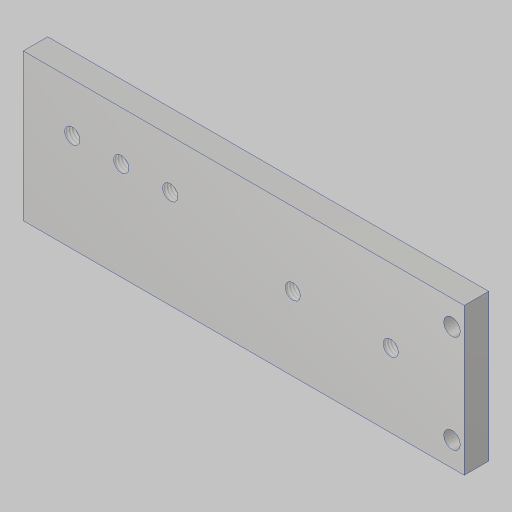
# Autodesk Inventor part: EL2-014
Saved by Autodesk Inventor 2023.5 (Build 275446000, 446)
## iProperties
Created: 2025-01-21
Part Number: EL2-014
Material: Aluminum 6061
Document SubType Name: Modeling
Designer: slick
Density: 2.7 g/cm^3
Appearance: Aluminum - Flat
Author: slick
Autodesk Inventor part; units mm, degrees
ref_plane "YZ Plane" through (0, 0, 0) normal (1, 0, 0) x (0, 1, 0)
ref_plane "XZ Plane" through (0, 0, 0) normal (0, 1, 0) x (-1, 0, 0)
ref_plane "XY Plane" through (0, 0, 0) normal (0, 0, 1) x (1, 0, 0)
sketch "Sketch1" plane through (0, 0, 0) normal (0, 0, 1) x (1, 0, 0)
  line L0 (57.15, -19.05) -> (-57.15, -19.05)
  line L1 (-57.15, -19.05) -> (-57.15, 19.05)
  line L2 (-57.15, 19.05) -> (57.15, 19.05)
  line L3 (57.15, 19.05) -> (57.15, -19.05)
  line L4 (57.15, -19.05) -> (-57.15, 19.05) construction
  line L5 (-57.15, -19.05) -> (57.15, 19.05) construction
  point P0 (0, 0)
  dimension "d0" = 114.3
  dimension "d1" = 38.1
  constraints: 12 end point, 2 midpoint, 2 parallel, 1 horizontal, 1 perpendicular
  measures "d0" distance of L1.end L2.end
  measures "d1" distance of L0.end L1.end
extrude "Extrusion1" add sketch "Sketch1" along normal blind 6.35
sketch "Sketch2" plane through (0, 0, 6.35) normal (0, 0, 1) x (1, 0, 0)
  line L0 (-57.15, 19.05) -> (-57.15, -19.05) projected
  line L1 (57.15, 19.05) -> (-57.15, 19.05) projected
  point P0 (0, 0)
  point P1 (-44.45, 6.35)
  point P2 (-31.75, 6.35)
  point P3 (-19.05, 6.35)
  point P4 (-57.15, 0)
  dimension "d5" = 12.7
  dimension "d6" = 12.7
  dimension "d14" = 12.7
  dimension "d15" = 12.7
  constraints: 2 horizontal alignment, 1 midpoint
  measures "d5" distance of point (-31.75, 6.35) point (-44.45, 6.35)
  measures "d6" distance of point (-31.75, 6.35) point (-19.05, 6.35)
  measures "d14" distance from line of L1 point (-44.45, 6.35)
  measures "d15" distance from line of L0 point (-44.45, 6.35)
hole "Hole1" at (-44.45, 6.35, 6.35) at (-31.75, 6.35, 6.35) at (-19.05, 6.35, 6.35) direction (0, 0, -1) diameter 3.9624 end through all thread size "10-32 UNF" class "2B" standard "ANSI Unified Screw Threads"
sketch "Sketch3" plane through (0, 0, 6.35) normal (0, 0, 1) x (1, 0, 0)
  line L0 (57.15, 19.05) -> (-57.15, 19.05) projected
  line L1 (-57.15, -19.05) -> (57.15, -19.05) projected
  line L2 (57.15, -19.05) -> (57.15, 19.05) projected
  point P0 (0, 0)
  point P1 (53.975, 12.7)
  point P2 (53.975, -12.7)
  dimension "d16" = 6.35
  dimension "d17" = 6.35
  dimension "d18" = 3.175
  constraints: 1 vertical alignment
  measures "d16" distance from line of L0 point (53.975, 12.7)
  measures "d17" distance from line of L1 point (53.975, -12.7)
  measures "d18" distance from line of L2 point (53.975, 12.7)
hole "Hole2" at (53.975, 12.7, 6.35) at (53.975, -12.7, 6.35) direction (0, 0, -1) diameter 4.318 end through all clearance for "Flat Head Machine Screw (82)" size "#8" standard "Ansi Unified Screw Threads"
sketch "Sketch5" plane through (0, 0, 6.35) normal (0, 0, 1) x (1, 0, 0)
  line L0 (57.15, -19.05) -> (57.15, 19.05) construction
  point P0 (0, 0)
  point P1 (12.7, 0)
  point P2 (38.1, 0)
  point P3 (57.15, 0)
  dimension "d28" = 25.4
  dimension "d29" = 19.05
  constraints: 2 horizontal alignment, 1 midpoint
  measures "d28" distance of point (38.1, 0) point (12.7, 0)
  measures "d29" distance from line of L0 point (38.1, 0)
hole "Hole3" at (12.7, 0, 6.35) at (38.1, 0, 6.35) direction (0, 0, -1) diameter 3.9624 end through all thread size "10-32 UNF" class "2B" standard "ANSI Unified Screw Threads"
equation "\"d5\" = d4"
equation "\"d6\" = d4"
equation "\"d4\" = 12.7"
body "Solid1"
